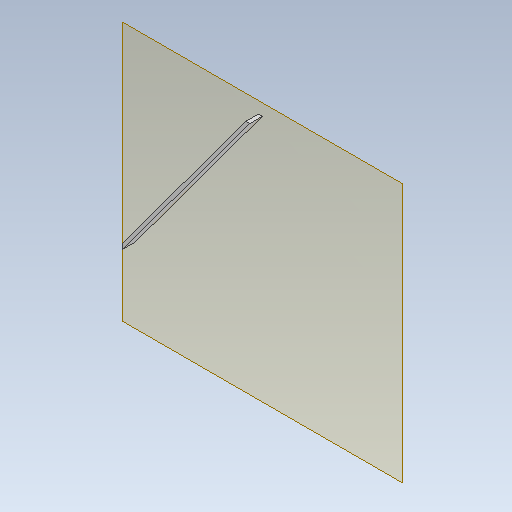
# Autodesk Inventor part: backWall
Saved by Autodesk Inventor 2021 (Build 250183000, 183)
## iProperties
Created: 2020-09-18
Part Number: backWall
Material: Generic
Document SubType Name: Modeling
Designer: deli
Density: 1 g/cm^3
Appearance: Default
Author: deli
Autodesk Inventor part; units mm, degrees
ref_plane "YZ Plane" through (0, 0, 0) normal (1, 0, 0) x (0, 1, 0)
ref_plane "XZ Plane" through (0, 0, 0) normal (0, 1, 0) x (-1, 0, 0)
ref_plane "XY Plane" through (0, 0, 0) normal (0, 0, 1) x (1, 0, 0)
ref_plane "Work Plane1" through (0, 0, 0) normal (0, 0, 1) x (1, 0, 0)
sketch "Sketch1" plane through (0, 0, 0) normal (0, 0, 1) x (1, 0, 0)
  line L0 (128.0033, 237.1649) -> (-128.0033, 237.1649) projected
  line L1 (-128.0033, 0) -> (-128.0033, 237.1649) projected
  line L2 (128.0033, 0) -> (-128.0033, 0) projected
  line L3 (128.0033, 237.1649) -> (128.0033, 0) projected
  line L4 (0, 237.1649) -> (-128.0033, 63.5)
  line L5 (-3.9443, 237.1649) -> (-128.0033, 68.8513)
  point P0 (0, 0)
  dimension "d0" = 63.5
  dimension "d1" = 128.0033
  dimension "d2" = 3.175
  constraints: 4 end point, 3 point on line, 1 midpoint, 1 parallel
  measures "d0" distance from line of L4.end L2
  measures "d1" distance from line of L3 L4.start
  measures "d2" distance between parallel lines of L4 L5
extrude "Extrusion1" add sketch "Sketch1" along normal blind 12.7 contours L4 L1 L5 L0
body "Solid1"
